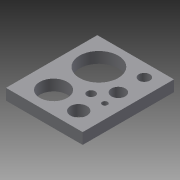
# Autodesk Inventor part: hole_test
Saved by Autodesk Inventor 2013 (Build 170138000, 138)
## iProperties
Created: 2013-06-22
Part Number: hole_test
Material: Generic
Document SubType Name: Modeling
Designer: Masta
Density: 1 g/cm^3
Author: Masta
Autodesk Inventor part; units mm, degrees
ref_plane "YZ Plane" through (0, 0, 0) normal (1, 0, 0) x (0, 1, 0)
ref_plane "XZ Plane" through (0, 0, 0) normal (0, 1, 0) x (-1, 0, 0)
ref_plane "XY Plane" through (0, 0, 0) normal (0, 0, 1) x (1, 0, 0)
sketch "Sketch1" plane through (0, 0, 0) normal (0, 0, 1) x (1, 0, 0)
  circle A0 centre (0, 0) radius 0.5
  circle A1 centre (-2.7681, 0.2813) radius 0.75
  circle A2 centre (-0.5, 7.6342) radius 1
  circle A3 centre (-0.5, 2.9376) radius 1.25
  circle A4 centre (-1.2054, -3.5313) radius 1.5
  circle A5 centre (-6.7502, -2.5313) radius 2.5
  circle A6 centre (-6.2681, 5.1832) radius 3.5
  line L0 (2.4912, -6.5091) -> (-11.3709, -6.5091)
  line L1 (-11.3709, -6.5091) -> (-11.3709, 10.0048)
  line L2 (-11.3709, 10.0048) -> (2.4912, 10.0048)
  line L3 (2.4912, 10.0048) -> (2.4912, -6.5091)
  dimension "d0" = 1
  dimension "d1" = 1.5
  dimension "d2" = 2
  dimension "d3" = 2.5
  dimension "d4" = 3
  dimension "d5" = 5
  dimension "d6" = 7
  constraints: 8 end point, 7 centre point, 2 parallel, 1 coincident, 1 horizontal, 1 perpendicular
  measures "d0" diameter of A0
  measures "d1" diameter of A1
  measures "d2" diameter of A2
  measures "d3" diameter of A3
  measures "d4" diameter of A4
  measures "d5" diameter of A5
  measures "d6" diameter of A6
extrude "Extrusion1" add sketch "Sketch1" along normal blind 2
body "Solid1"
